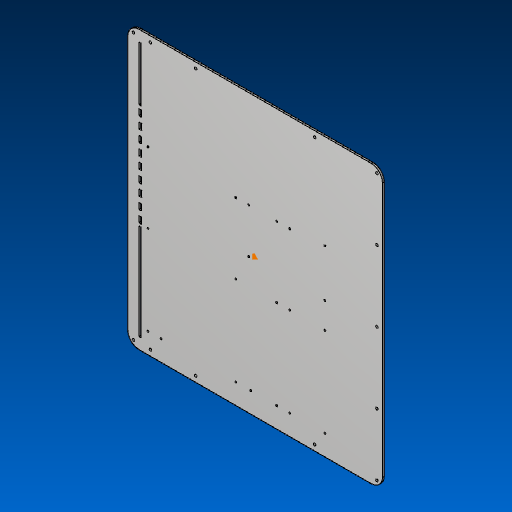
# Autodesk Inventor part: right_panel
Saved by Autodesk Inventor 2018 (Build 220112000, 112)
## iProperties
Created: 2019-10-14
Part Number: right_panel
Material: アルミニウム 6061
Document SubType Name: Modeling
Designer: gisen
Density: 2.7 g/cm^3
Appearance: アルミニウム - フラット
Author: gisen
Autodesk Inventor part; units mm, degrees
ref_plane "YZ Plane" through (0, 0, 0) normal (1, 0, 0) x (0, 1, 0)
ref_plane "XZ Plane" through (0, 0, 0) normal (0, 1, 0) x (-1, 0, 0)
ref_plane "XY Plane" through (0, 0, 0) normal (0, 0, 1) x (1, 0, 0)
sketch "スケッチ1" plane through (0, 0, 0) normal (0, 0, 1) x (1, 0, 0)
  line L0 (-205, -245) -> (205, -245)
  line L1 (225, -225) -> (225, 225)
  line L2 (205, 245) -> (-205, 245)
  line L3 (-225, 225) -> (-225, -225)
  line L4 (-225, -245) -> (225, 245) construction
  line L5 (225, -245) -> (-225, 245) construction
  circle A0 centre (-215, 235) radius 2.25
  circle A1 centre (215, 235) radius 2.25
  circle A2 centre (-215, -235) radius 2.25
  circle A3 centre (215, -235) radius 2.25
  arc A4 (-205, 245) -> (-225, 225) centre (-205, 225) ccw
  arc A5 (225, 225) -> (205, 245) centre (205, 225) ccw
  arc A6 (205, -245) -> (225, -225) centre (205, -225) ccw
  arc A7 (-225, -225) -> (-205, -245) centre (-205, -225) ccw
  point P0 (0, 0)
  dimension "d0" = 450
  dimension "d1" = 490
  dimension "d2" = 4.5
  dimension "d3" = 10
  dimension "d4" = 10
  dimension "d5" = 10
  dimension "d6" = 10
  dimension "d7" = 10
  dimension "d8" = 10
  dimension "d9" = 10
  dimension "d10" = 10
  dimension "d11" = 20
  constraints: 12 end point, 8 centre point, 8 point on circle, 8 point on line, 8 tangent, 6 equal radius, 2 midpoint, 2 parallel, 1 horizontal, 1 perpendicular
  measures "d0" distance of L5.end L4.end
  measures "d1" distance of L4.end L5.start
  measures "d2" diameter of A0
  measures "d3" distance from line of A0.centre L2
  measures "d4" distance from line of L3 A0.centre
  measures "d5" distance from line of A1.centre L2
  measures "d6" distance from line of L1 A1.centre
  measures "d7" distance from line of L1 A3.centre
  measures "d8" distance from line of L0 A3.centre
  measures "d9" distance from line of L0 A2.centre
  measures "d10" distance from line of L3 A2.centre
  measures "d11" radius of A4
extrude "押し出し1" add sketch "スケッチ1" along normal blind 3
sketch "スケッチ2" plane through (0, 0, 3) normal (0, 0, 1) x (1, 0, 0)
  circle A0 centre (38.092, 72.9258) radius 1.6
  circle A1 centre (-34.298, 72.9258) radius 1.6
  circle A2 centre (-189.238, 72.9258) radius 1.6
  circle A3 centre (-189.238, -51.5342) radius 1.6
  circle A4 centre (-166.378, -209.0142) radius 1.6
  circle A5 centre (-34.298, -209.0142) radius 1.6
  circle A6 centre (38.092, -209.0142) radius 1.6
  circle A7 centre (38.092, -51.5342) radius 1.6
  circle A8 centre (-34.298, -51.5342) radius 1.6
  circle A9 centre (38.092, -209.0142) radius 2.25 projected
  circle A10 centre (-166.378, -209.0142) radius 2.25 projected
  circle A11 centre (38.092, -51.5342) radius 2.25 projected
  circle A12 centre (38.092, 72.9258) radius 2.25 projected
  circle A13 centre (-34.298, -209.0142) radius 2.25 projected
  circle A14 centre (-34.298, -51.5342) radius 2.25 projected
  circle A15 centre (-34.298, 72.9258) radius 2.25 projected
  circle A16 centre (-189.238, -51.5342) radius 2.25 projected
  circle A17 centre (-189.238, 72.9258) radius 2.25 projected
  point P0 (0, 0)
  dimension "d14" = 3.2
  constraints: 9 centre point, 9 concentric, 8 equal radius
  measures "d14" diameter of A0
extrude "押し出し2" cut sketch "スケッチ2" against normal blind 3 contours A0 | A1 | A2 | A3 | A4 | A5 | A6 | A7 | A8
sketch "スケッチ4" plane through (0, 0, 3) normal (0, 0, 1) x (1, 0, 0)
  line L0 (-205, -225) -> (-202, -225) projected
  line L1 (-205, -30.5483) -> (-205, -20.2613) projected
  line L2 (-205, -30.5483) -> (-202, -30.5483) projected
  line L3 (-202, -20.2613) -> (-202, -30.5483) projected
  line L4 (-205, -20.2613) -> (-202, -20.2613) projected
  line L5 (-205, -9.8937) -> (-205, 0.3933) projected
  line L6 (-205, -9.8937) -> (-202, -9.8937) projected
  line L7 (-202, 0.3933) -> (-202, -9.8937) projected
  line L8 (-205, 0.3933) -> (-202, 0.3933) projected
  line L9 (-205, 10.4517) -> (-205, 20.7387) projected
  line L10 (-205, 10.4517) -> (-202, 10.4517) projected
  line L11 (-202, 20.7387) -> (-202, 10.4517) projected
  line L12 (-205, 20.7387) -> (-202, 20.7387) projected
  line L13 (-205, 31.1063) -> (-205, 41.3933) projected
  line L14 (-205, 31.1063) -> (-202, 31.1063) projected
  line L15 (-202, 41.3933) -> (-202, 31.1063) projected
  line L16 (-205, 41.3933) -> (-202, 41.3933) projected
  line L17 (-205, 51.4517) -> (-205, 61.7387) projected
  line L18 (-205, 51.4517) -> (-202, 51.4517) projected
  line L19 (-202, 61.7387) -> (-202, 51.4517) projected
  line L20 (-205, 61.7387) -> (-202, 61.7387) projected
  line L21 (-205, 72.1063) -> (-205, 82.3933) projected
  line L22 (-205, 72.1063) -> (-202, 72.1063) projected
  line L23 (-202, 82.3933) -> (-202, 72.1063) projected
  line L24 (-205, 82.3933) -> (-202, 82.3933) projected
  line L25 (-205, 92.4517) -> (-205, 102.7387) projected
  line L26 (-205, 92.4517) -> (-202, 92.4517) projected
  line L27 (-202, 102.7387) -> (-202, 92.4517) projected
  line L28 (-205, 102.7387) -> (-202, 102.7387) projected
  line L29 (-205, 225) -> (-205, 129.6) projected
  line L30 (-205, 129.6) -> (-202, 129.6) projected
  line L31 (-202, 225) -> (-202, 129.6) projected
  line L32 (-205, 225) -> (-202, 225) projected
  line L33 (-202, 102.7387) -> (-201, 102.7387)
  line L34 (-201, 102.7387) -> (-201, 92.4517)
  line L35 (-201, 92.4517) -> (-202, 92.4517)
  line L36 (-202, 82.3933) -> (-201, 82.3933)
  line L37 (-201, 82.3933) -> (-201, 72.1063)
  line L38 (-201, 72.1063) -> (-202, 72.1063)
  line L39 (-202, 61.7387) -> (-201, 61.7387)
  line L40 (-201, 61.7387) -> (-201, 51.4517)
  line L41 (-201, 51.4517) -> (-202, 51.4517)
  line L42 (-202, 41.3933) -> (-201, 41.3933)
  line L43 (-201, 41.3933) -> (-201, 31.1063)
  line L44 (-201, 31.1063) -> (-202, 31.1063)
  line L45 (-202, 20.7387) -> (-201, 20.7387)
  line L46 (-201, 20.7387) -> (-201, 10.4517)
  line L47 (-201, 10.4517) -> (-202, 10.4517)
  line L48 (-202, 0.3933) -> (-201, 0.3933)
  line L49 (-201, 0.3933) -> (-201, -9.8937)
  line L50 (-201, -9.8937) -> (-202, -9.8937)
  line L51 (-202, -20.2613) -> (-201, -20.2613)
  line L52 (-201, -20.2613) -> (-201, -30.5483)
  line L53 (-201, -30.5483) -> (-202, -30.5483)
  line L54 (-202, -40.6067) -> (-201, -40.6067)
  line L55 (-201, -40.6067) -> (-201, -50.8937)
  line L56 (-201, -50.8937) -> (-202, -50.8937)
  line L57 (-205, -225) -> (-205, -56.0642) projected
  line L58 (-202, -56.0642) -> (-202, -225) projected
  line L59 (-205, 112.7971) -> (-202, 112.7971) projected
  line L60 (-205, 123.0841) -> (-205, 112.7971) projected
  line L61 (-205, 123.0841) -> (-202, 123.0841) projected
  line L62 (-202, 112.7971) -> (-201, 112.7971)
  line L63 (-201, 112.7971) -> (-201, 123.0841)
  line L64 (-201, 123.0841) -> (-202, 123.0841)
  line L65 (-202, -40.6067) -> (-202, -50.8937) construction
  line L66 (-202, -50.8937) -> (-205, -50.8937)
  line L67 (-205, -50.8937) -> (-205, -40.6067)
  line L68 (-205, -40.6067) -> (-202, -40.6067)
  line L69 (-205, -56.0642) -> (-202, -56.0642) projected
  point P0 (0, 0)
  point P1 (-225, -58.3552)
  point P2 (-222, -58.3552)
  point P3 (-225, -120.4005)
  point P4 (-222, -120.4005)
  dimension "d17" = 1
  constraints: 60 end point, 17 perpendicular, 10 equal length, 10 horizontal, 2 collinear, 4 other
  measures "d17" distance of L27.start L33.end
extrude "押し出し3" cut sketch "スケッチ4" against normal blind 3
sketch "スケッチ5" plane through (0, 0, 3) normal (0, 0, 1) x (1, 0, 0)
  circle A0 centre (-215, 235) radius 2.25 construction
  circle A1 centre (-215, -235) radius 2.25 construction
  circle A2 centre (-185, -235) radius 2.25
  line L0 (-205, -245) -> (205, -245) projected
  circle A3 centre (-185, 235) radius 2.25
  line L1 (205, 245) -> (-205, 245) projected
  point P0 (0, 0)
  dimension "d20" = 30
  dimension "d21" = 10
  dimension "d22" = 30
  dimension "d23" = 10
  constraints: 2 centre point, 2 equal radius
  measures "d20" distance of A1.centre A2.centre
  measures "d21" distance from line of L0 A2.centre
  measures "d22" distance of A0.centre A3.centre
  measures "d23" distance from line of L1 A3.centre
extrude "押し出し4" cut sketch "スケッチ5" against normal blind 3
sketch "スケッチ7" plane through (0, 0, 3) normal (0, 0, 1) x (1, 0, 0)
  line L0 (225, 225) -> (225, -225) projected
  circle A0 centre (-105, -235) radius 2.25 projected
  circle A1 centre (215, 0) radius 2.25 projected
  circle A2 centre (105, -235) radius 2.25 projected
  circle A3 centre (215, 125) radius 2.25 projected
  circle A4 centre (-105, 235) radius 2.25 projected
  circle A5 centre (-215, -125) radius 2.25 projected
  circle A6 centre (-215, 0) radius 2.25 projected
  circle A7 centre (105, 235) radius 2.25 projected
  circle A8 centre (215, -125) radius 2.25 projected
  line L1 (-205.2, 132.4) -> (-201.8, 132.4) projected
  line L2 (-201.8, 132.4) -> (-201.8, 225.2) projected
  line L3 (-201.8, 225.2) -> (-205.2, 225.2) projected
  circle A9 centre (215, 235) radius 2.25 projected
  circle A10 centre (-215, 235) radius 2.25 projected
  circle A11 centre (215, -235) radius 2.25 projected
  circle A12 centre (-215, -235) radius 2.25 projected
  line L4 (205, -245) -> (-205, -245) projected
  arc A13 (-225, -225) -> (-205, -245) centre (-205, -225) ccw projected
  line L5 (-225, -225) -> (-225, 225) projected
  arc A14 (-205, 245) -> (-225, 225) centre (-205, 225) ccw projected
  line L6 (-205, 245) -> (205, 245) projected
  arc A15 (225, 225) -> (205, 245) centre (205, 225) ccw projected
  line L7 (225, 225) -> (225, -225) projected
  arc A16 (205, -245) -> (225, -225) centre (205, -225) ccw projected
  line L8 (-205.2, 225.2) -> (-205.2, 132.4) projected
  circle A17 centre (-215, 125) radius 2.25 projected
  point P0 (0, 0)
extrude "押し出し6" cut sketch "スケッチ7" against normal up to surface (3 mm away) contours A0 | A1 | A2 | A3 | A4 | A7 | A8
sketch "スケッチ8" plane through (0, 0, 0) normal (0, 0, -1) x (-1, 0, 0)
  line L0 (-49.775, 130.075) -> (-150.225, 130.075) construction
  line L1 (-150.225, 130.075) -> (-150.225, 199.925) construction
  line L2 (-150.225, 199.925) -> (-49.775, 199.925) construction
  line L3 (-49.775, 199.925) -> (-49.775, 130.075) construction
  line L4 (-49.775, 130.075) -> (-150.225, 199.925) construction
  line L5 (-150.225, 130.075) -> (-49.775, 199.925) construction
  line L6 (205, 245) -> (-205, 245) construction
  line L7 (-225, 225) -> (-225, -225) construction
  line L8 (-59.625, 195.86) -> (-136.225, 195.86) construction
  line L9 (-136.225, 195.86) -> (-136.225, 134.14) construction
  line L10 (-136.225, 134.14) -> (-59.625, 134.14) construction
  line L11 (-59.625, 134.14) -> (-59.625, 195.86) construction
  line L12 (-59.625, 195.86) -> (-136.225, 134.14) construction
  line L13 (-136.225, 195.86) -> (-59.625, 134.14) construction
  line L14 (-97.925, 165) -> (-100, 165) construction
  circle A0 centre (-59.625, 134.14) radius 1.6
  circle A1 centre (-59.625, 195.86) radius 1.6
  circle A2 centre (-136.225, 195.86) radius 1.6
  circle A3 centre (-136.225, 134.14) radius 1.6
  point P0 (0, 0)
  dimension "d40" = 69.85
  dimension "d41" = 100.45
  dimension "d42" = 80
  dimension "d43" = 125
  dimension "d44" = 61.72
  dimension "d45" = 90.6
  dimension "d46" = 14
  dimension "d47" = 3.2
  dimension "d48" = 3.2
  dimension "d49" = 3.2
  dimension "d50" = 3.2
  constraints: 26 end point, 4 centre point, 4 coincident, 4 midpoint, 4 parallel, 3 horizontal, 2 perpendicular
  measures "d40" distance of L0.end L1.end
  measures "d41" distance of L0.start L0.end
  measures "d42" distance from line of L6 L14.end
  measures "d43" distance from line of L7 L14.end
  measures "d44" distance of L10.end L8.start
  measures "d45" distance between parallel lines of L1 L11
  measures "d46" distance between parallel lines of L1 L9
  measures "d47" diameter of A0
  measures "d48" diameter of A1
  measures "d49" diameter of A2
  measures "d50" diameter of A3
extrude "押し出し7" [suppressed]
sketch "スケッチ9" plane through (0, 0, 0) normal (0, 0, -1) x (-1, 0, 0)
  circle A0 centre (166.378, -209.0142) radius 1.6 construction
  circle A1 centre (34.298, -209.0142) radius 1.6 construction
  circle A2 centre (-38.092, -209.0142) radius 1.6 construction
  circle A3 centre (189.238, -51.5342) radius 1.6 construction
  circle A4 centre (189.238, 72.9258) radius 1.6 construction
  circle A5 centre (34.298, 72.9258) radius 1.6 construction
  circle A6 centre (-38.092, 72.9258) radius 1.6 construction
  circle A7 centre (34.298, -51.5342) radius 1.6 construction
  circle A8 centre (-38.092, -51.5342) radius 1.6 construction
  line L0 (199.398, -215.3642) -> (-72.382, -215.3642) construction
  line L1 (-72.382, -215.3642) -> (-72.382, 89.4358) construction
  line L2 (-72.382, 89.4358) -> (199.398, 89.4358) construction
  line L3 (199.398, 89.4358) -> (199.398, -215.3642) construction
  point P0 (0, 0)
  dimension "d53" = 6.35
  dimension "d54" = 33.02
  dimension "d55" = 304.8
  dimension "d56" = 271.78
  constraints: 8 end point, 2 parallel, 1 horizontal, 1 perpendicular
  measures "d53" distance from line of A0.centre L0
  measures "d54" distance from line of L3 A0.centre
  measures "d55" distance of L2.end L0.start
  measures "d56" distance of L0.start L0.end
sketch "スケッチ10" plane through (0, 0, 0) normal (0, 0, -1) x (-1, 0, 0)
  line L0 (199.398, -215.3642) -> (-130.802, -215.3642) construction
  line L1 (-130.802, -215.3642) -> (-130.802, 89.4358) construction
  line L2 (-130.802, 89.4358) -> (199.398, 89.4358) construction
  line L3 (199.398, 89.4358) -> (199.398, -215.3642) construction
  circle A0 centre (189.238, 72.9258) radius 1.6 construction
  circle A1 centre (-215, -125) radius 2.25 projected
  circle A2 centre (-123.182, 78.0058) radius 1.6
  circle A3 centre (189.238, 72.9258) radius 1.6 construction
  line L4 (189.238, 72.9258) -> (34.298, 72.9258) construction
  circle A4 centre (34.298, 72.9258) radius 1.6 construction
  circle A5 centre (34.298, 72.9258) radius 1.6 construction
  line L5 (34.298, 72.9258) -> (-38.092, 72.9258) construction
  line L6 (-38.092, 72.9258) -> (-60.952, 72.9258) construction
  circle A6 centre (-38.092, 72.9258) radius 1.6
  circle A7 centre (-60.952, 72.9258) radius 1.6
  line L7 (-123.182, 78.0058) -> (-123.182, -5.8142) construction
  line L8 (-123.182, -5.8142) -> (-123.182, -51.5342) construction
  line L9 (-123.182, -51.5342) -> (-123.182, -208.9142) construction
  circle A8 centre (-123.182, -5.8142) radius 1.6
  circle A9 centre (-123.182, -51.5342) radius 1.6
  circle A10 centre (-123.182, -208.9142) radius 1.6
  line L10 (-123.182, -5.8142) -> (11.438, -5.8142) construction
  circle A11 centre (11.438, -5.8142) radius 1.6
  line L11 (11.438, -5.8142) -> (11.438, 72.9258) construction
  circle A12 centre (11.438, 72.9258) radius 1.6
  line L12 (189.238, 72.9258) -> (189.238, -209.0142) construction
  circle A13 centre (166.378, -209.0142) radius 1.6 construction
  line L13 (189.238, -209.0142) -> (166.378, -209.0142) construction
  circle A14 centre (189.238, -209.0142) radius 1.6
  line L14 (-60.952, 72.9258) -> (-60.952, -209.0142) construction
  line L15 (-60.952, -209.0142) -> (-38.092, -209.0142) construction
  circle A15 centre (-38.092, -51.5342) radius 1.6 construction
  line L16 (-38.092, -51.5342) -> (-60.952, -51.5342) construction
  circle A16 centre (-38.092, -209.0142) radius 1.6 construction
  circle A17 centre (-60.952, -51.5342) radius 1.6
  circle A18 centre (-60.952, -209.0142) radius 1.6
  line L17 (-38.092, -209.0142) -> (166.378, -209.0142) construction
  circle A19 centre (7.628, -209.0142) radius 1.6
  point P0 (0, 0)
  dimension "d57" = 330.2
  dimension "d58" = 304.8
  dimension "d59" = 10.16
  dimension "d60" = 16.51
  dimension "d61" = 84.198
  dimension "d62" = 5.08
  dimension "d63" = 312.42
  dimension "d64" = 154.94
  dimension "d65" = 227.33
  dimension "d66" = 250.19
  dimension "d67" = 78.74
  dimension "d68" = 124.46
  dimension "d69" = 281.84
  dimension "d70" = 177.8
  dimension "d71" = 134.62
  dimension "d72" = 16.51
  dimension "d73" = 181.61
  dimension "d74" = 3.2
  constraints: 36 end point, 14 centre point, 13 coincident, 13 equal radius, 6 point on line, 5 horizontal, 4 perpendicular, 4 vertical, 2 parallel
  measures "d57" distance of L0.start L0.end
  measures "d58" distance of L0.end L1.end
  measures "d59" distance from line of A0.centre L3
  measures "d60" distance from line of L2 A0.centre
  measures "d61" distance from line of L1 A1.centre
  measures "d62" vertical distance of A0.centre L7.start
  measures "d63" horizontal distance of A0.centre L7.start
  measures "d64" distance of L4.start L4.end
  measures "d65" distance of L5.end L4.start
  measures "d66" distance of L4.start L6.end
  measures "d67" vertical distance of L10.start A0.centre
  measures "d68" vertical distance of L8.end A0.centre
  measures "d69" vertical distance of L4.start L9.end
  measures "d70" horizontal distance of L4.start L10.end
  measures "d71" distance of L10.start L10.end
  measures "d72" distance from line of L2 L11.end
  measures "d73" distance from line of L12 A19.centre
  measures "d74" diameter of A0
extrude "押し出し8" cut sketch "スケッチ10" against normal blind 10 contours A2 | A7 | A8 | A9 | A10 | A11 | A12 | A14 | A17 | A18 | A19
sketch "スケッチ11" plane through (0, 0, 3) normal (0, 0, 1) x (1, 0, 0)
  point P0 (0, 0)
sketch "スケッチ12" plane through (0, 0, 0) normal (0, 0, -1) x (-1, 0, 0)
  line L0 (202, 225) -> (205, 225) construction
  line L1 (202, 129.6) -> (202, 225) construction
  line L2 (205, 225) -> (205, 129.6) construction
  line L3 (205, 129.6) -> (202, 129.6) construction
  line L4 (201, 123.0841) -> (205, 123.0841) construction
  line L5 (201, 112.7971) -> (201, 123.0841) construction
  line L6 (205, 123.0841) -> (205, 112.7971) construction
  line L7 (205, 112.7971) -> (201, 112.7971) construction
  line L8 (201, 102.7387) -> (205, 102.7387) construction
  line L9 (205, 102.7387) -> (205, 92.4517) construction
  line L10 (205, 92.4517) -> (201, 92.4517) construction
  line L11 (201, 92.4517) -> (201, 102.7387) construction
  line L12 (201, 82.3933) -> (205, 82.3933) construction
  line L13 (205, 82.3933) -> (205, 72.1063) construction
  line L14 (205, 72.1063) -> (201, 72.1063) construction
  line L15 (201, 72.1063) -> (201, 82.3933) construction
  line L16 (201, 61.7387) -> (205, 61.7387) construction
  line L17 (201, 51.4517) -> (201, 61.7387) construction
  line L18 (205, 51.4517) -> (201, 51.4517) construction
  line L19 (205, 61.7387) -> (205, 51.4517) construction
  line L20 (201, 41.3933) -> (205, 41.3933) construction
  line L21 (201, 31.1063) -> (201, 41.3933) construction
  line L22 (205, 31.1063) -> (201, 31.1063) construction
  line L23 (205, 41.3933) -> (205, 31.1063) construction
  line L24 (201, 20.7387) -> (205, 20.7387) construction
  line L25 (201, 10.4517) -> (201, 20.7387) construction
  line L26 (205, 10.4517) -> (201, 10.4517) construction
  line L27 (205, 20.7387) -> (205, 10.4517) construction
  line L28 (201, 0.3933) -> (205, 0.3933) construction
  line L29 (201, -9.8937) -> (201, 0.3933) construction
  line L30 (205, -9.8937) -> (201, -9.8937) construction
  line L31 (205, 0.3933) -> (205, -9.8937) construction
  line L32 (201, -20.2613) -> (205, -20.2613) construction
  line L33 (201, -30.5483) -> (201, -20.2613) construction
  line L34 (205, -30.5483) -> (201, -30.5483) construction
  line L35 (205, -20.2613) -> (205, -30.5483) construction
  line L36 (201, -40.6067) -> (205, -40.6067) construction
  line L37 (201, -50.8937) -> (201, -40.6067) construction
  line L38 (205, -50.8937) -> (201, -50.8937) construction
  line L39 (205, -40.6067) -> (205, -50.8937) construction
  line L40 (202, -56.0642) -> (205, -56.0642) construction
  line L41 (202, -225) -> (202, -56.0642) construction
  line L42 (205, -56.0642) -> (205, -225) construction
  line L43 (205, -225) -> (202, -225) construction
  line L44 (201.8, -225.2) -> (201.8, -55.8642)
  line L45 (201.8, -55.8642) -> (205.2, -55.8642)
  line L46 (205.2, -55.8642) -> (205.2, -225.2)
  line L47 (205.2, -225.2) -> (201.8, -225.2)
  line L48 (205.2, -51.0937) -> (200.8, -51.0937)
  line L49 (200.8, -51.0937) -> (200.8, -40.4067)
  line L50 (200.8, -40.4067) -> (205.2, -40.4067)
  line L51 (205.2, -40.4067) -> (205.2, -51.0937)
  line L52 (200.8, -30.7483) -> (200.8, -20.0613)
  line L53 (200.8, -20.0613) -> (205.2, -20.0613)
  line L54 (205.2, -20.0613) -> (205.2, -30.7483)
  line L55 (205.2, -30.7483) -> (200.8, -30.7483)
  line L56 (200.8, -10.0937) -> (200.8, 0.5933)
  line L57 (200.8, 0.5933) -> (205.2, 0.5933)
  line L58 (205.2, 0.5933) -> (205.2, -10.0937)
  line L59 (205.2, -10.0937) -> (200.8, -10.0937)
  line L60 (200.8, 10.2517) -> (200.8, 20.9387)
  line L61 (200.8, 20.9387) -> (205.2, 20.9387)
  line L62 (205.2, 20.9387) -> (205.2, 10.2517)
  line L63 (205.2, 10.2517) -> (200.8, 10.2517)
  line L64 (205.2, 30.9063) -> (200.8, 30.9063)
  line L65 (200.8, 30.9063) -> (200.8, 41.5933)
  line L66 (200.8, 41.5933) -> (205.2, 41.5933)
  line L67 (205.2, 41.5933) -> (205.2, 30.9063)
  line L68 (200.8, 51.2517) -> (200.8, 61.9387)
  line L69 (200.8, 61.9387) -> (205.2, 61.9387)
  line L70 (205.2, 61.9387) -> (205.2, 51.2517)
  line L71 (205.2, 51.2517) -> (200.8, 51.2517)
  line L72 (200.8, 71.9063) -> (205.2, 71.9063)
  line L73 (205.2, 71.9063) -> (205.2, 82.5933)
  line L74 (205.2, 82.5933) -> (200.8, 82.5933)
  line L75 (200.8, 82.5933) -> (200.8, 71.9063)
  line L76 (200.8, 92.2517) -> (205.2, 92.2517)
  line L77 (205.2, 92.2517) -> (205.2, 102.9387)
  line L78 (205.2, 102.9387) -> (200.8, 102.9387)
  line L79 (200.8, 102.9387) -> (200.8, 92.2517)
  line L80 (200.8, 112.5971) -> (200.8, 123.2841)
  line L81 (200.8, 123.2841) -> (205.2, 123.2841)
  line L82 (205.2, 123.2841) -> (205.2, 112.5971)
  line L83 (205.2, 112.5971) -> (200.8, 112.5971)
  line L84 (201.8, 129.4) -> (201.8, 225.2)
  line L85 (201.8, 225.2) -> (205.2, 225.2)
  line L86 (205.2, 225.2) -> (205.2, 129.4)
  line L87 (205.2, 129.4) -> (201.8, 129.4)
  point P0 (0, 0)
  dimension "d17" = 1
  dimension "d128" = 0.2
  dimension "d129" = 0.2
  dimension "d130" = 0.2
  dimension "d131" = 0.2
  dimension "d132" = 0.2
  dimension "d133" = 0.2
  dimension "d134" = 0.2
  dimension "d135" = 0.2
  dimension "d136" = 0.2
  dimension "d137" = 0.2
  dimension "d138" = 0.2
  constraints: 88 end point, 33 other
  measures "d128" distance between parallel lines of L43 L47
  measures "d129" distance between parallel lines of L39 L51
  measures "d130" distance between parallel lines of L34 L55
  measures "d131" distance between parallel lines of L30 L59
  measures "d132" distance between parallel lines of L26 L63
  measures "d133" distance between parallel lines of L23 L67
  measures "d134" distance between parallel lines of L18 L71
  measures "d135" distance between parallel lines of L14 L72
  measures "d136" distance between parallel lines of L10 L76
  measures "d137" distance between parallel lines of L7 L83
  measures "d138" distance between parallel lines of L3 L87
extrude "押し出し9" cut sketch "スケッチ12" against normal through all
equation "\"d5\" = d3"
equation "\"d6\" = d4"
equation "\"d7\" = d6"
equation "\"d8\" = d5"
equation "\"d9\" = d8"
equation "\"d10\" = d7"
